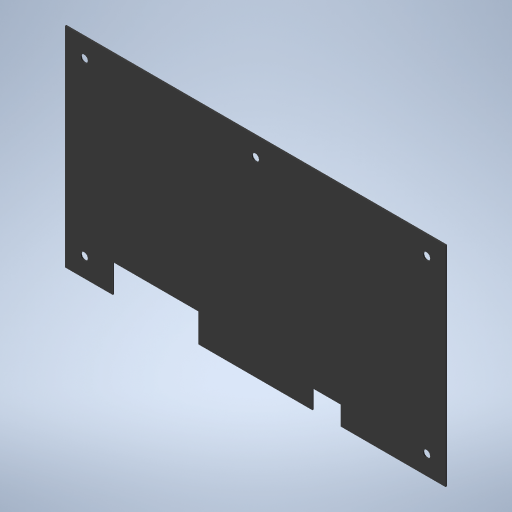
# Autodesk Inventor part: Top Intake Poly (Sponsor Panel)
Saved by Autodesk Inventor 2023 (Build 270158000, 158)
## iProperties
Created: 2024-02-16
Part Number: Top Intake Poly (Sponsor Panel)
Material: Generic
Document SubType Name: Modeling
Designer: Robodox
Density: 1 g/cm^3
Appearance: Default
Author: Robodox
Autodesk Inventor part; units mm, degrees
ref_plane "YZ Plane" through (0, 0, 0) normal (1, 0, 0) x (0, 1, 0)
ref_plane "XZ Plane" through (0, 0, 0) normal (0, 1, 0) x (-1, 0, 0)
ref_plane "XY Plane" through (0, 0, 0) normal (0, 0, 1) x (1, 0, 0)
sketch "Sketch1" plane through (0, 0, 0) normal (0, 0, 1) x (1, 0, 0)
  line L0 (-125.8778, 76.6863) -> (128.1222, 76.6863)
  line L1 (128.1222, 76.6863) -> (128.1222, -63.0137)
  line L2 (128.1222, -63.0137) -> (-125.8778, -63.0137)
  line L3 (-125.8778, -63.0137) -> (-125.8778, 76.6863)
  line L4 (-125.8778, -63.0137) -> (-94.1278, -63.0137)
  line L5 (-94.1278, -63.0137) -> (-94.1278, -43.9637)
  line L6 (-94.1278, -43.9637) -> (-36.9778, -43.9637)
  line L7 (-36.9778, -43.9637) -> (-36.9778, -63.0137)
  line L8 (128.1222, -63.0137) -> (58.2722, -63.0137)
  line L9 (58.2722, -63.0137) -> (58.2722, -50.3137)
  line L10 (58.2722, -50.3137) -> (39.2222, -50.3137)
  line L11 (39.2222, -50.3137) -> (39.2222, -63.0137)
  line L12 (-125.8778, 76.6863) -> (-113.1778, 76.6863)
  line L13 (-113.1778, 76.6863) -> (-113.1778, 63.9863)
  circle A0 centre (-113.1778, 63.9863) radius 2.54
  line L14 (-113.1778, 63.9863) -> (1.1222, 63.9863)
  circle A1 centre (1.1222, 63.9863) radius 2.54
  line L15 (1.1222, 63.9863) -> (115.4222, 63.9863)
  circle A2 centre (115.4222, 63.9863) radius 2.54
  line L16 (-125.8778, -63.0137) -> (-113.1778, -63.0137)
  line L17 (-113.1778, -63.0137) -> (-113.1778, -50.3137)
  circle A3 centre (-113.1778, -50.3137) radius 2.54
  line L18 (128.1222, -63.0137) -> (128.1222, -50.3137)
  line L19 (128.1222, -50.3137) -> (115.4222, -50.3137)
  circle A4 centre (115.4222, -50.3137) radius 2.54
  point P0 (0, 0)
  dimension "d0" = 254
  dimension "d1" = 139.7
  dimension "d6" = 31.75
  dimension "d7" = 19.05
  dimension "d8" = 57.15
  dimension "d9" = 69.85
  dimension "d10" = 12.7
  dimension "d11" = 19.05
  dimension "d14" = 12.7
  dimension "d15" = 12.7
  dimension "d16" = 5.08
  dimension "d17" = 114.3
  dimension "d18" = 5.08
  dimension "d19" = 114.3
  dimension "d20" = 5.08
  dimension "d21" = 12.7
  dimension "d22" = 12.7
  dimension "d23" = 5.08
  dimension "d24" = 12.7
  dimension "d25" = 12.7
  dimension "d26" = 5.08
  constraints: 40 end point, 10 perpendicular, 7 point on line, 5 centre point, 5 coincident, 3 horizontal, 2 parallel
  measures "d0" distance of L0.start L0.end
  measures "d1" distance of L0.end L1.end
  measures "d6" distance of L2.end L4.end
  measures "d7" distance of L4.end L5.end
  measures "d8" distance of L5.end L6.end
  measures "d9" distance of L1.end L8.end
  measures "d10" distance of L8.end L9.end
  measures "d11" distance of L9.end L10.end
  measures "d14" distance of L0.start L12.end
  measures "d15" distance of L12.end L13.end
  measures "d16" diameter of A0
  measures "d17" distance of L14.start L14.end
  measures "d18" diameter of A1
  measures "d19" distance of L15.start L15.end
  measures "d20" diameter of A2
  measures "d21" distance of L2.end L16.end
  measures "d22" distance of L16.end L17.end
  measures "d23" diameter of A3
  measures "d24" distance of L1.end L18.end
  measures "d25" distance of L18.end L19.end
  measures "d26" diameter of A4
extrude "Extrusion4" add sketch "Sketch1" along normal blind 0.7937 contours L0 L1 L2 L9 L10 L11 L7 L6 L5 L3
body "Solid4"
